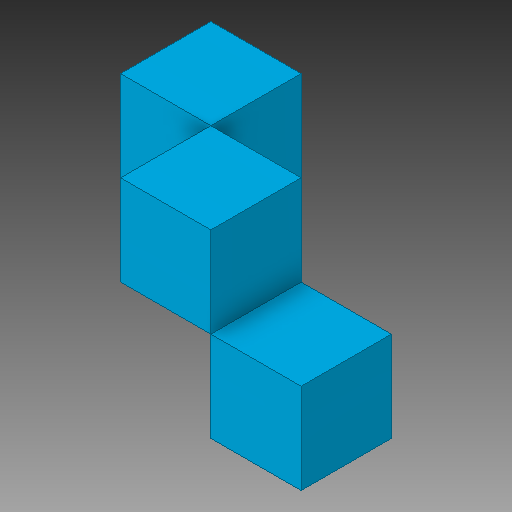
# Autodesk Inventor part: Light Blue Part
Saved by Autodesk Inventor 2018 (Build 220112000, 112)
## iProperties
Created: 2017-11-15
Part Number: Light Blue Part
Material: Wood (Maple)
Document SubType Name: Modeling
Designer: 232963
Density: 0.67 g/cm^3
Appearance: Sky Blue Medium
Mass: 18.5276 g
Surface Area: 79.8385 cm^2
Volume: 27.6532 cm^3
Author: 232963
Autodesk Inventor part; units mm, degrees
ref_plane "YZ Plane" through (0, 0, 0) normal (1, 0, 0) x (0, 1, 0)
ref_plane "XZ Plane" through (0, 0, 0) normal (0, 1, 0) x (-1, 0, 0)
ref_plane "XY Plane" through (0, 0, 0) normal (0, 0, 1) x (1, 0, 0)
sketch "Sketch1" plane through (0, 0, 0) normal (0, 0, 1) x (1, 0, 0)
  line L0 (-0.7054, 38.1) -> (18.3446, 38.1)
  line L1 (18.3446, 38.1) -> (18.3446, 0)
  line L2 (18.3446, 0) -> (-0.7054, 0)
  line L3 (-0.7054, 0) -> (-0.7054, 38.1)
  point P0 (0, 0)
  dimension "d0" = 38.1
  dimension "d1" = 19.05
  constraints: 8 end point, 2 parallel, 1 horizontal, 1 perpendicular
  measures "d0" distance of L0.end L1.end
  measures "d1" distance of L1.end L2.end
extrude "Extrusion1" add sketch "Sketch1" along normal blind 19.05
sketch "Sketch2" plane through (0, 0, 19.05) normal (0, 0, 1) x (1, 0, 0)
  line L0 (18.3446, 0) -> (18.3446, 38.1) projected
  line L1 (18.3446, 38.1) -> (37.3946, 38.1)
  line L2 (37.3946, 38.1) -> (37.3946, 19.05)
  line L3 (37.3946, 19.05) -> (18.3446, 19.05)
  line L4 (18.3446, 19.05) -> (18.3446, 38.1)
  point P0 (0, 0)
  dimension "d4" = 19.05
  dimension "d5" = 19.05
  constraints: 8 end point, 2 parallel, 1 horizontal, 1 perpendicular
  measures "d4" distance of L2.end L3.end
  measures "d5" distance of L1.end L2.end
extrude "Extrusion2" add sketch "Sketch2" along normal blind 19.05
sketch "Sketch3" plane through (18.3446, 19.05, 19.05) normal (0, -1, 0) x (1, 0, 0)
  line L0 (19.05, 0) -> (19.05, 19.05) projected
  line L1 (19.05, 19.05) -> (38.1, 19.05)
  line L2 (38.1, 19.05) -> (38.1, 0)
  line L3 (38.1, 0) -> (19.05, 0)
  line L4 (19.05, 0) -> (19.05, 19.05)
  point P0 (-18.3446, -19.05)
  dimension "d8" = 19.05
  dimension "d9" = 19.05
  constraints: 8 end point, 2 parallel, 1 horizontal, 1 perpendicular
  measures "d8" distance of L2.end L3.end
  measures "d9" distance of L1.end L2.end
extrude "Extrusion3" add sketch "Sketch3" along normal blind 19.05
body "Solid1"
